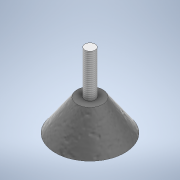
# Autodesk Inventor part: Pata regulable M6
Saved by Autodesk Inventor 2020 (Build 240168000, 168)
## iProperties
Created: 2020-05-20
Part Number: Pata regulable M6
Material: Genérico
Document SubType Name: Modeling
Designer: Leon
Density: 1 g/cm^3
Appearance: Valor por defecto
Mass: 11.5572 g
Surface Area: 41.3028 cm^2
Volume: 11.5572 cm^3
Author: Leon
Autodesk Inventor part; units mm, degrees
ref_plane "YZ Plane" through (0, 0, 0) normal (1, 0, 0) x (0, 1, 0)
ref_plane "XZ Plane" through (0, 0, 0) normal (0, 1, 0) x (-1, 0, 0)
ref_plane "XY Plane" through (0, 0, 0) normal (0, 0, 1) x (1, 0, 0)
sketch "Boceto1" plane through (0, 0, 0) normal (0, 1, 0) x (-1, 0, 0)
  circle A0 centre (0, 0) radius 20
  circle A1 centre (0, 0) radius 3
  dimension "d0" = 40
  dimension "d1" = 6
  constraints: 2 centre point, 2 coincident
  measures "d0" diameter of A0
  measures "d1" diameter of A1
extrude "Extrusión1" add sketch "Boceto1" along normal blind 25 contours A1
extrude "Extrusión2" add sketch "Boceto1" against normal blind 18
draft "Cara para el ángulo de desmoldeo1" angle -35 pull direction (0, -1, 0) faces at (-19.9351, -12, -1.6093) fixed edges at (20, -18, 0)
thread "Rosca1" size "M6x1" class "6g" standard "ANSI Metric M Profile" full length
